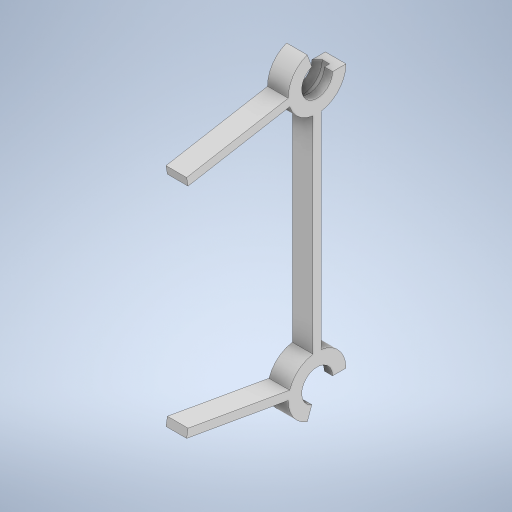
# Autodesk Inventor part: lens mounts
Saved by Autodesk Inventor 2024 (Build 280153000, 153)
## iProperties
Created: 2025-01-15
Part Number: lens mounts
Material: Generic
Document SubType Name: Modeling
Designer: Williamow
Density: 1 g/cm^3
Appearance: Default
Author: Williamow
Autodesk Inventor part; units mm, degrees
ref_plane "Work Plane1" through (-2, 20, -2.8) normal (0, -1, 0) x (1, 0, 0)
ref_plane "YZ Plane" through (0, 0, 0) normal (1, 0, 0) x (0, 1, 0)
ref_plane "XZ Plane" through (0, 0, 0) normal (0, 1, 0) x (-1, 0, 0)
sketch "Sketch1" plane through (0, 0, 0) normal (0, 1, 0) x (-1, 0, 0)
  line L0 (2, -1.5) -> (1.5, -2)
  line L1 (1.5, -2) -> (0.79, -2)
  line L2 (0.79, -2) -> (0.79, -1.5)
  line L3 (0.79, -1.5) -> (0, -1.5)
  line L4 (0, -1.5) -> (0, -2.8)
  line L5 (0, -2.8) -> (2, -2.8)
  line L6 (2, -2.8) -> (2, -1.5)
  line L7 (0, 0) -> (1.5115, 0)
  line L8 (2, -12.5) -> (2, -13.8)
  line L9 (2, -13.8) -> (0, -13.8)
  line L10 (0, -13.8) -> (0, -12.5)
  line L11 (0, -12.5) -> (0.5, -13)
  line L12 (0.5, -13) -> (1.5, -13)
  line L13 (1.5, -13) -> (2, -12.5)
  line L14 (0, -10) -> (1, -10)
  point P0 (1, -13)
  dimension "d0" = 0.5
  dimension "d1" = 45
  dimension "d2" = 0.8
  dimension "d3" = 0.71
  dimension "d5" = 2
  dimension "d6" = 1
  dimension "d7" = 0.8
  dimension "d8" = 0.5
  dimension "d9" = 10
  dimension "d10" = 3
  constraints: 30 end point, 8 perpendicular, 4 vertical alignment, 3 horizontal, 2 equal length, 1 horizontal alignment, 1 midpoint, 1 parallel, 1 vertical
  measures "d0" distance of L1.end L2.end
  measures "d1" angle of L6 L0
  measures "d2" distance from line of L5 L1.end
  measures "d3" distance of L0.end L1.end
  measures "d5" distance between parallel lines of L7 L1
  measures "d6" distance of L11.end L12.end
  measures "d7" distance between parallel lines of L9 L12
  measures "d8" distance from line of L8.start L12
  measures "d9" distance of L14.start L7.start
  measures "d10" distance between parallel lines of L14 L12
revolve "Revolution1" add sketch "Sketch1" angle 250 about axis through (0, 0, 0) along (1, 0, 0) contours L6 L5 L4 L3 L2 L1 L0
sketch "Sketch3" plane through (-2, 0, -2.8) normal (-1, 0, 0) x (0, 0, 1)
  arc A0 (3.7577, -2.6311) -> (0, 0) centre (2.8, 0) ccw projected
  line L0 (2.4, 2.7713) -> (2.4, 12.7713)
  line L1 (2.4, 12.7713) -> (3.2, 12.7713)
  line L2 (3.2, 12.7713) -> (3.2, 2.7713)
  line L3 (5.4597, 0.8752) -> (15.3078, 2.6116)
  line L4 (15.3078, 2.6116) -> (15.4467, 1.8238)
  line L5 (15.4467, 1.8238) -> (5.5986, 0.0873)
  point P0 (2.8, 0)
  dimension "d31" = 0.8
  dimension "d32" = 10
  dimension "d33" = 80
  dimension "d14" = 0.81
  dimension "d16" = 2
  dimension "d18" = 2
  dimension "d19" = 0.81
  dimension "d20" = 70
  dimension "d27" = 1.356
  dimension "d28" = 0.8
  constraints: 12 end point, 4 equal length, 4 perpendicular, 4 point on circle, 1 vertical
  measures "d31" distance of L0.end L1.end
  measures "d32" distance of L1.end L2.end
  measures "d33" angle of L3 L2
extrude "Extrusion4" add sketch "Sketch3" against normal up to surface (2 mm away)
mirror "Mirror3" about plane through (-2, 12.7713, -0.4) normal (0, 1, 0) of "Extrusion4", "Revolution1"
body "Solid1"
